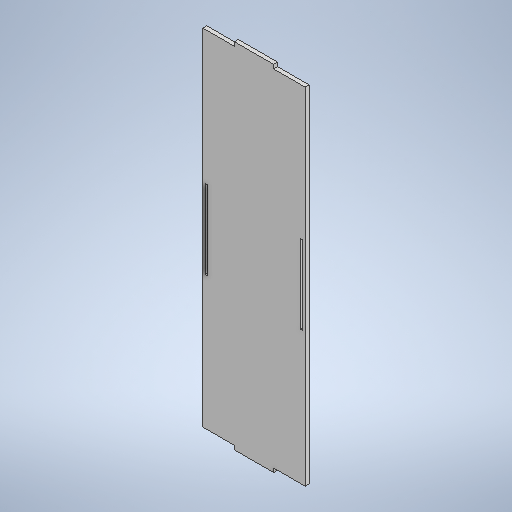
# Autodesk Inventor part: Part1
Saved by Autodesk Inventor 2025.4 (Build 294407000, 407)
## iProperties
Created: 2026-05-23
Part Number: Part1
Material: Generic
Document SubType Name: Modeling
Designer: lenovo
Density: 1 g/cm^3
Appearance: Default
Author: lenovo
Autodesk Inventor part; units mm, degrees
ref_plane "YZ Plane" through (0, 0, 0) normal (1, 0, 0) x (0, 1, 0)
ref_plane "XZ Plane" through (0, 0, 0) normal (0, 1, 0) x (-1, 0, 0)
ref_plane "XY Plane" through (0, 0, 0) normal (0, 0, 1) x (1, 0, 0)
sketch "Sketch1" plane through (0, 0, 0) normal (0, 0, 1) x (1, 0, 0)
  line L0 (-65, -219.5) -> (65, -219.5)
  line L1 (65, -219.5) -> (65, 219.5)
  line L2 (65, 219.5) -> (-65, 219.5)
  line L3 (-65, 219.5) -> (-65, -219.5)
  line L4 (-65, -219.5) -> (65, 219.5) construction
  line L5 (65, -219.5) -> (-65, 219.5) construction
  line L6 (58.93, -50) -> (62, -50)
  line L7 (62, -50) -> (62, 50)
  line L8 (62, 50) -> (58.93, 50)
  line L9 (58.93, 50) -> (58.93, -50)
  line L10 (58.93, -50) -> (62, 50) construction
  line L11 (62, -50) -> (58.93, 50) construction
  line L12 (0, 219.5) -> (0, -219.5)
  line L13 (-58.93, -50) -> (-62, -50)
  line L14 (-62, -50) -> (-62, 50)
  line L15 (-62, 50) -> (-58.93, 50)
  line L16 (-58.93, 50) -> (-58.93, -50)
  line L17 (-58.93, -50) -> (-62, 50) construction
  line L18 (-62, -50) -> (-58.93, 50) construction
  point P0 (0, 0)
  point P1 (60.465, 0)
  point P2 (62, 0)
  point P3 (-60.465, 0)
  point P4 (-62, 0)
  point P5 (0, 0)
  dimension "d0" = 130
  dimension "d1" = 439
  dimension "d2" = 3.07
  dimension "d3" = 100
  dimension "d4" = 3
  constraints: 38 end point, 8 midpoint, 6 symmetric about line, 4 parallel, 2 horizontal, 2 perpendicular, 1 horizontal alignment
  measures "d0" distance of L2.end L1.end
  measures "d1" distance of L0.end L1.end
  measures "d2" distance of L8.end L7.end
  measures "d3" distance of L7.end L6.end
  measures "d4" distance from line of L1 point (62, 0)
extrude "Extrusion1" add sketch "Sketch1" along normal mid plane 5
sketch "Sketch2" plane through (0, 0, 2.5) normal (0, 0, 1) x (1, 0, 0)
  line L0 (-25, 219.5) -> (25, 219.5)
  line L1 (25, 219.5) -> (25, 224.5)
  line L2 (25, 224.5) -> (-25, 224.5)
  line L3 (-25, 224.5) -> (-25, 219.5)
  line L4 (-58.93, -50) -> (-58.93, 50) projected
  line L5 (-58.93, 0) -> (58.93, 0)
  line L6 (58.93, -50) -> (58.93, 50) projected
  line L7 (-25, -219.5) -> (25, -219.5)
  line L8 (25, -219.5) -> (25, -224.5)
  line L9 (25, -224.5) -> (-25, -224.5)
  line L10 (-25, -224.5) -> (-25, -219.5)
  point P0 (0, 0)
  point P1 (-65, 219.5)
  point P2 (0, 224.5)
  point P3 (0, -224.5)
  dimension "d7" = 50
  dimension "d8" = 5
  constraints: 18 end point, 5 symmetric about line, 3 midpoint, 2 parallel, 1 horizontal, 1 horizontal alignment, 1 perpendicular, 1 vertical alignment
  measures "d7" distance of L1.end L2.end
  measures "d8" distance of L0.end L1.end
extrude "Extrusion2" add sketch "Sketch2" against normal blind 5
body "Solid1"
